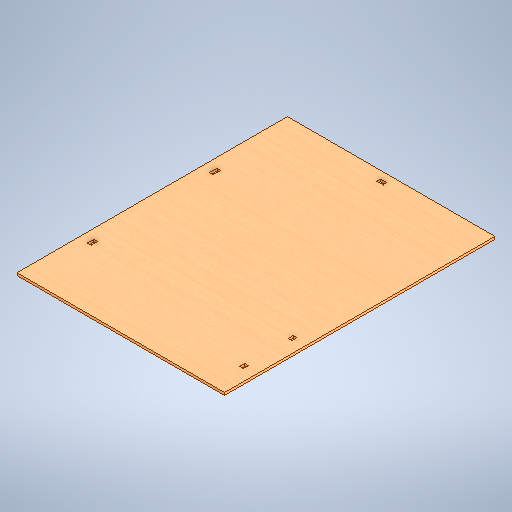
# Autodesk Inventor part: MainFloorPanel
Saved by Autodesk Inventor 2026.2 (Build 302298010, 298A)
## iProperties
Created: 2026-03-17
Part Number: MainFloorPanel
Material: Drewno (wiśnia)
Document SubType Name: Modeling
Designer: Patryk
Density: 0.63 g/cm^3
Appearance: Wiśnia — naturalna — niski połysk
Mass: 301.518 g
Surface Area: 2452.04 cm^2
Volume: 478.6 cm^3
Author: Patryk
Autodesk Inventor part; units mm, degrees
ref_plane "YZ Plane" through (0, 0, 0) normal (1, 0, 0) x (0, 1, 0)
ref_plane "XZ Plane" through (0, 0, 0) normal (0, 1, 0) x (-1, 0, 0)
ref_plane "XY Plane" through (0, 0, 0) normal (0, 0, 1) x (1, 0, 0)
sketch "Szkic1" plane through (0, 0, 0) normal (0, 1, 0) x (-1, 0, 0)
  line L0 (-165, -215) -> (165, -215)
  line L1 (165, -215) -> (165, 215)
  line L2 (165, 215) -> (-165, 215)
  line L3 (-165, 215) -> (-165, -215)
  line L4 (-165, -215) -> (165, 215) construction
  line L5 (165, -215) -> (-165, 215) construction
  point P0 (0, 0)
  dimension "d0" = 330
  dimension "d1" = 430
  constraints: 12 end point, 2 midpoint, 2 parallel, 1 horizontal, 1 perpendicular
  measures "d0" distance of L2.end L1.end
  measures "d1" distance of L1.end L0.end
extrude "Wyciągnięcie proste1" add sketch "Szkic1" along normal mid plane 4
sketch "Szkic2" plane through (0, 2, 0) normal (0, 1, 0) x (1, 0, 0)
  line L0 (165, -215) -> (165, 215) projected
  line L1 (-165, -215) -> (165, -215) projected
  line L2 (165, 215) -> (-165, 215) projected
  line L3 (147, -159) -> (141, -159)
  line L4 (141, -159) -> (141, -167)
  line L5 (141, -167) -> (147, -167)
  line L6 (147, -167) -> (147, -159)
  line L7 (147, -82) -> (141, -82)
  line L8 (141, -82) -> (141, -90)
  line L9 (141, -90) -> (147, -90)
  line L10 (147, -90) -> (147, -82)
  line L11 (-165, 215) -> (-165, -215) projected
  line L12 (-150, -118) -> (-144, -118)
  line L13 (-144, -118) -> (-144, -108)
  line L14 (-144, -108) -> (-150, -108)
  line L15 (-150, -108) -> (-150, -118)
  line L16 (-150, 76) -> (-144, 76)
  line L17 (-144, 76) -> (-144, 88)
  line L18 (-144, 88) -> (-150, 88)
  line L19 (-150, 88) -> (-150, 76)
  line L20 (5, 197) -> (-5, 197)
  line L21 (-5, 197) -> (-5, 203)
  line L22 (-5, 203) -> (5, 203)
  line L23 (5, 203) -> (5, 197)
  point P0 (0, 0)
  dimension "d39" = 48
  dimension "d40" = 6
  dimension "d41" = 18
  dimension "d42" = 8
  dimension "d43" = 125
  dimension "d44" = 8
  dimension "d45" = 18
  dimension "d46" = 6
  dimension "d59" = 6
  dimension "d60" = 10
  dimension "d61" = 15
  dimension "d62" = 97
  dimension "d65" = 6
  dimension "d66" = 12
  dimension "d67" = 15
  dimension "d68" = 127
  dimension "d71" = 12
  dimension "d72" = 6
  dimension "d73" = 160
  dimension "d74" = 10
  constraints: 40 end point, 10 parallel, 5 horizontal, 5 perpendicular
  measures "d39" distance between parallel lines of L1 L5
  measures "d40" distance of L3.start L3.end
  measures "d41" distance between parallel lines of L0 L6
  measures "d42" distance of L3.end L4.end
  measures "d43" distance between parallel lines of L1 L9
  measures "d44" distance of L7.end L8.end
  measures "d45" distance between parallel lines of L10 L0
  measures "d46" distance of L7.start L7.end
  measures "d59" distance of L14.end L13.end
  measures "d60" distance of L13.end L12.end
  measures "d61" distance from line of L12.start L11
  measures "d62" distance between parallel lines of L12 L1
  measures "d65" distance of L18.end L17.end
  measures "d66" distance of L17.end L16.end
  measures "d67" distance from line of L16.start L11
  measures "d68" distance between parallel lines of L2 L18
  measures "d71" distance between parallel lines of L2 L22
  measures "d72" distance of L20.end L21.end
  measures "d73" distance between parallel lines of L0 L23
  measures "d74" distance of L20.start L20.end
extrude "Wyciągnięcie proste7" cut sketch "Szkic2" against normal through all contours L6 L5 L4 L3 | L10 L9 L8 L7 | L15 L14 L13 L12
extrude "Wyciągnięcie proste8" cut sketch "Szkic2" against normal through all contours L19 L18 L17 L16
extrude "Wyciągnięcie proste9" cut sketch "Szkic2" against normal through all contours L20 L21 L22 L23
